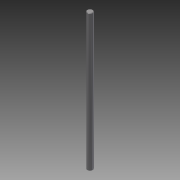
# Autodesk Inventor part: 6mmx150mmSmoothRod
Saved by Autodesk Inventor 2014 SP1 (Build 180222100, 222)
## iProperties
Created: 2016-11-27
Part Number: 6mmx150mmSmoothRod
Material: Generic
Document SubType Name: Modeling
Designer: danielsikar
Density: 1 g/cm^3
Appearance: Stainless - Brushed
Author: danielsikar
Autodesk Inventor part; units mm, degrees
ref_plane "YZ Plane" through (0, 0, 0) normal (1, 0, 0) x (0, 1, 0)
ref_plane "XZ Plane" through (0, 0, 0) normal (0, 1, 0) x (-1, 0, 0)
ref_plane "XY Plane" through (0, 0, 0) normal (0, 0, 1) x (1, 0, 0)
sketch "Sketch1" plane through (0, 0, 0) normal (0, 0, 1) x (1, 0, 0)
  circle A0 centre (0, 0) radius 3
  dimension "d0" = 6
  constraints: 1 centre point, 1 coincident
  measures "d0" diameter of A0
extrude "Extrusion1" add sketch "Sketch1" along normal blind 150
chamfer "Chamfer1" distance 0.5 angle 45 1 edges at (-3, 0, 0)
chamfer "Chamfer2" distance 0.5 angle 45 1 edges at (-3, 0, 150)
body "Solid1"
